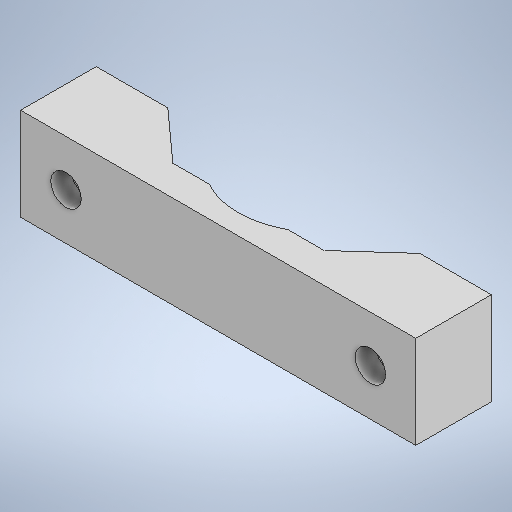
# Autodesk Inventor part: CameraTopSlider
Saved by Autodesk Inventor 2025.1 (Build 291241000, 241)
## iProperties
Created: 2026-04-27
Part Number: CameraTopSlider
Material: Generic
Document SubType Name: Modeling
Designer: User
Density: 1 g/cm^3
Appearance: Default
Author: User
## iProperties of the stored document CameraTopSlider_3DPrint.ipt
Created: 2026-04-30
Part Number: CameraTopSlider_3DPrint
Material: Generic
Document SubType Name: Modeling
Designer: User
Density: 1 g/cm^3
Appearance: Default
Author: User
Autodesk Inventor part; units mm, degrees
ref_plane "YZ Plane" through (0, 0, 0) normal (1, 0, 0) x (0, 1, 0)
ref_plane "XZ Plane" through (0, 0, 0) normal (0, 1, 0) x (-1, 0, 0)
ref_plane "XY Plane" through (0, 0, 0) normal (0, 0, 1) x (1, 0, 0)
sketch "Sketch1" plane through (0, 0, 0) normal (0, 0, 1) x (1, 0, 0)
  line L0 (-0.2, 0) -> (25.2, 0) projected
  line L1 (25.4, -1) -> (29.8, -1) projected
  line L2 (30, -0.8) -> (30, 3.8) projected
  line L3 (29.8, 4) -> (25.4, 4) projected
  line L4 (25.2, 3) -> (-0.2, 3) projected
  line L5 (-0.4, 4) -> (-4.8, 4) projected
  line L6 (-5, 3.8) -> (-5, -0.8) projected
  line L7 (-4.8, -1) -> (-0.4, -1) projected
  line L8 (25.1, -0.1) -> (-0.1, -0.1)
  line L9 (-0.1, -0.1) -> (-0.1, -1.1)
  line L10 (-0.1, -1.1) -> (-5.1, -1.1)
  line L11 (-5.1, -1.1) -> (-5.1, 4.1)
  line L12 (-5.1, 4.1) -> (-0.1, 4.1)
  line L13 (-0.1, 4.1) -> (-0.1, 3.1)
  line L14 (-0.1, 3.1) -> (25.1, 3.1)
  line L15 (25.1, 3.1) -> (25.1, 4.1)
  line L16 (25.1, 4.1) -> (30.1, 4.1)
  line L17 (30.1, 4.1) -> (30.1, -1.1)
  line L18 (30.1, -1.1) -> (25.1, -1.1)
  line L19 (25.1, -1.1) -> (25.1, -0.1)
  circle A0 centre (27.6, 1.5) radius 1.4 projected
  circle A1 centre (-2.6, 1.5) radius 1.4 projected
  line L20 (25.4, -1) -> (25.2, -0.8) projected
  line L21 (30, -0.8) -> (29.8, -1) projected
  line L22 (29.8, 4) -> (30, 3.8) projected
  line L23 (25.2, 3.8) -> (25.4, 4) projected
  line L24 (-0.4, 4) -> (-0.2, 3.8) projected
  line L25 (-5, 3.8) -> (-4.8, 4) projected
  line L26 (-4.8, -1) -> (-5, -0.8) projected
  line L27 (-0.2, -0.8) -> (-0.4, -1) projected
  line L28 (25.2, 3.8) -> (25.2, 3) projected
  line L29 (-0.2, 3) -> (-0.2, 3.8) projected
  line L30 (-0.2, -0.8) -> (-0.2, 0) projected
  line L31 (25.2, 0) -> (25.2, -0.8) projected
  point P0 (0, 0)
  dimension "d0" = 0.1
  constraints: 24 end point, 4 other
  measures "d0" distance between parallel lines of L0 L8
extrude "Extrusion1" add sketch "Sketch1" along normal blind 2 contours L30 L27 L7 L26 L6 L25 L5 L24 L29 L4 L28 L23 L3 L22 L2 L21 L1 L20 L31 L0 | L8 L9 L10 L11 L12 L13 L14 L15 L16 L17 L18 L19 | A0 | A1
sketch "Sketch2" plane through (0, 0, 2) normal (0, 0, 1) x (1, 0, 0)
  line L0 (25.1, -1.1) -> (30.1, -1.1) projected
  line L1 (30.1, -1.1) -> (30.1, 4.1) projected
  line L2 (30.1, 4.1) -> (25.1, 4.1) projected
  line L3 (25.1, 4.1) -> (25.1, 3.1) projected
  line L4 (25.1, 3.1) -> (-0.1, 3.1) projected
  line L5 (-0.1, 3.1) -> (-0.1, 4.1) projected
  line L6 (-0.1, 4.1) -> (-5.1, 4.1) projected
  line L7 (-5.1, 4.1) -> (-5.1, -1.1) projected
  line L8 (-5.1, -1.1) -> (-0.1, -1.1) projected
  line L9 (-0.1, -1.1) -> (-0.1, -0.1) projected
  line L10 (-0.1, -0.1) -> (25.1, -0.1) projected
  line L11 (25.1, -0.1) -> (25.1, -1.1) projected
  line L12 (-7.1, 6.1) -> (1.9, 6.1)
  line L13 (1.9, 6.1) -> (1.9, 5.1)
  line L14 (1.9, 5.1) -> (23.1, 5.1)
  line L15 (23.1, 5.1) -> (23.1, 6.1)
  line L16 (23.1, 6.1) -> (32.1, 6.1)
  line L17 (32.1, 6.1) -> (32.1, -3.1)
  line L18 (32.1, -3.1) -> (23.1, -3.1)
  line L19 (23.1, -3.1) -> (23.1, -2.1)
  line L20 (23.1, -2.1) -> (1.9, -2.1)
  line L21 (1.9, -2.1) -> (1.9, -3.1)
  line L22 (1.9, -3.1) -> (-7.1, -3.1)
  line L23 (-7.1, -3.1) -> (-7.1, 6.1)
  point P0 (0, 0)
  dimension "d3" = 2
  constraints: 24 end point, 11 other
  measures "d3" distance between parallel lines of L6 L12
ref_plane "Work Plane1" through (22.5, -3.5, -5.5) normal (0, 0, -1) x (0, 1, 0)
extrude "Extrusion2" add sketch "Sketch2" against normal up to surface (7.5 mm away)
sketch "Sketch3" plane through (1.9, -2.1, 2) normal (0, -1, 0) x (1, 0, 0)
  line L0 (6.9944, -4) -> (4.1, -4) projected
  arc A0 (8.2059, -3.4222) -> (6.9944, -4) centre (10.6, -10) ccw projected
  arc A1 (10.6, -3) -> (8.2059, -3.4222) centre (10.6, -10) ccw projected
  arc A2 (10.6, -3) -> (8.2059, -3.4222) centre (10.6, -10) ccw projected
  arc A3 (12.9941, -3.4222) -> (10.6, -3) centre (10.6, -10) ccw projected
  circle A4 centre (10.6, -10) radius 5.6 projected
  arc A5 (14.2056, -4) -> (12.9941, -3.4222) centre (10.6, -10) ccw projected
  line L1 (17.1, -4) -> (14.2056, -4) projected
  line L2 (17.1, -7.4019) -> (17.1, -4) projected
  line L3 (4.1, -4) -> (4.1, -7.4019) projected
  circle A6 centre (10.6, -10) radius 5.6 projected
  arc A7 (4.1, -7.4019) -> (3.8918, -8) centre (10.6, -10) ccw projected
  arc A8 (17.3082, -8) -> (17.1, -7.4019) centre (10.6, -10) ccw projected
  arc A9 (7.8638, -2.4825) -> (6.727, -3) centre (10.6, -10) ccw
  line L4 (6.727, -3) -> (3.1, -3)
  line L5 (3.1, -3) -> (3.1, -7.2161)
  arc A10 (3.1, -7.2161) -> (2.9335, -7.7143) centre (10.6, -10) ccw
  arc A11 (10.6, -2) -> (7.8638, -2.4825) centre (10.6, -10) ccw
  arc A12 (13.3362, -2.4825) -> (10.6, -2) centre (10.6, -10) ccw
  arc A13 (14.473, -3) -> (13.3362, -2.4825) centre (10.6, -10) ccw
  line L6 (14.473, -3) -> (18.1, -3)
  line L7 (18.1, -3) -> (18.1, -7.2161)
  arc A14 (18.2665, -7.7143) -> (18.1, -7.2161) centre (10.6, -10) ccw
  line L8 (0, -7.5) -> (21.2, -7.5) projected
  point P0 (-1.9, -2)
  point P1 (17.1383, -7.5)
  point P2 (18.1993, -7.5)
  point P3 (10.6, -2)
  point P4 (7.8638, -2.4825)
  point P5 (3.0007, -7.5)
  point P6 (4.0617, -7.5)
  dimension "d6" = 1
  dimension "d7" = 1
  dimension "d8" = 1
  constraints: 12 point on circle, 8 end point, 6 centre point, 7 other
  measures "d6" radial gap between concentric circles of A0 A9
  measures "d7" radial gap between concentric circles of A1 A11
  measures "d8" radial gap between concentric circles of A3 A12
extrude "Extrusion3" cut sketch "Sketch3" against normal blind 10 contours A0 A1 A3 A5 L1 L2 A8 L8 A4 A7 L3 L0 | L0 L3 A7 L8 A10 L5 L4 A9 A11 A12 A13 L6 L7 A14 A8 L2 L1 A5 A3 A1 A0 | A4 L8 picked at (9.9261, -6.5925)
sketch "Sketch4" plane through (1.9, -2.1, 2) normal (0, -1, 0) x (1, 0, 0)
  line L0 (3.1, -7.2161) -> (3.1, -3) projected
  line L1 (0, -7.5) -> (3.0007, -7.5) projected
  line L2 (-9, -7.5) -> (0, -7.5) projected
  line L3 (-1.9, -6.3) -> (-1.9, -15) projected
  line L4 (18.1, -3) -> (18.1, -7.2161) projected
  arc A0 (3.1, -7.2161) -> (3.0007, -7.5) centre (10.6, -10) ccw projected
  arc A1 (18.1993, -7.5) -> (18.1, -7.2161) centre (10.6, -10) ccw projected
  line L5 (18.1993, -7.5) -> (21.2, -7.5) projected
  line L6 (21.2, -7.5) -> (30.2, -7.5) projected
  line L7 (23.1, -15) -> (23.1, -6.3) projected
  line L8 (3.1, -3) -> (-1.9, -7.5)
  line L9 (18.1, -3) -> (14.473, -3) projected
  line L10 (18.1, -3) -> (23.1, -7.5)
  point P0 (-1.9, -2)
  constraints: 4 end point, 4 point on line
extrude "Extrusion4" cut sketch "Sketch4" along normal mid plane 33.75
sketch "Sketch5" plane through (0, 0, 2) normal (0, 0, 1) x (1, 0, 0)
  line L0 (-2, -1) -> (-4.8, -1) projected
  line L1 (-5, -0.8) -> (-5, 3.8) projected
  line L2 (-4.8, 4) -> (-2, 4) projected
  line L3 (27, 4) -> (29.8, 4) projected
  line L4 (30, 3.8) -> (30, -0.8) projected
  line L5 (29.8, -1) -> (27, -1) projected
  line L6 (25.2, 4) -> (30, -1)
  line L7 (-0.2, 4) -> (-5, -1)
  circle A0 centre (-2.6, 1.5) radius 1.5
  circle A1 centre (27.6, 1.5) radius 1.5
  line L8 (30, 3.8) -> (29.8, 4) projected
  line L9 (29.8, -1) -> (30, -0.8) projected
  line L10 (-5, -0.8) -> (-4.8, -1) projected
  line L11 (-4.8, 4) -> (-5, 3.8) projected
  arc A2 (-2, 2.7649) -> (-2, 0.2351) centre (-2.6, 1.5) ccw projected
  line L12 (-2, 2.7649) -> (-2, 4) projected
  line L13 (-2, -1) -> (-2, 0.2351) projected
  arc A3 (27, 0.2351) -> (27, 2.7649) centre (27.6, 1.5) ccw projected
  line L14 (27, 0.2351) -> (27, -1) projected
  line L15 (27, 4) -> (27, 2.7649) projected
  dimension "d13" = 3
  dimension "d14" = 3
  constraints: 4 end point, 2 centre point, 2 midpoint
  measures "d13" diameter of A0
  measures "d14" diameter of A1
extrude "Extrusion5" cut sketch "Sketch5" against normal blind 33.75 contours L13 A2 L7 A0 | A0 L7 A2 L13 | A0 L12 A2 L7 | A2 L12 A0 L7 | L15 A3 L6 A1 | A1 L6 A3 L15 | L6 A3 L14 A1 | A1 L14 A3 L6
chamfer "Chamfer1" distance 0.2 angle 45 4 edges at (25.1, 3.1, -2.75) (25.1, -0.1, -2.75) (-0.1, -0.1, -2.75) (-0.1, 3.1, -2.75)
sketch "Sketch6" plane through (16.373, 3.1, -1) normal (0, -1, 0) x (1, 0, 0)
  line L0 (8.527, 1) -> (8.527, -4.41) projected
  line L1 (8.527, 1) -> (-3.873, 1) projected
  arc A0 (0, 0) -> (-3.873, 1) centre (-3.873, -7) ccw projected
  line L2 (0, 0) -> (3.627, 0) projected
  line L3 (3.627, 0) -> (8.527, -4.41) projected
  line L4 (8.627, -4.5) -> (8.727, -4.5) projected
  line L5 (8.727, -4.5) -> (8.727, 1) projected
  line L6 (8.727, 1) -> (8.527, 1) projected
  line L7 (8.527, 1) -> (8.527, -4.41) projected
  line L8 (8.527, -4.41) -> (8.627, -4.5) projected
  line L9 (8.727, 1) -> (8.727, -4.5) projected
  line L10 (-16.273, -4.41) -> (-16.273, 1) projected
  line L11 (-16.273, -4.41) -> (-11.373, 0) projected
  line L12 (-11.373, 0) -> (-7.746, 0) projected
  arc A1 (-3.873, 1) -> (-7.746, 0) centre (-3.873, -7) ccw projected
  line L13 (-3.873, 1) -> (-16.273, 1) projected
  line L14 (-16.373, -4.5) -> (-16.273, -4.41) projected
  line L15 (-16.273, -4.41) -> (-16.273, 1) projected
  line L16 (-16.273, 1) -> (-16.473, 1) projected
  line L17 (-16.473, 1) -> (-16.473, -4.5) projected
  line L18 (-16.473, -4.5) -> (-16.373, -4.5) projected
  point P0 (-16.373, 1)
  point P1 (-3.873, 1)
  point P2 (-3.873, 1)
  point P3 (-3.873, 1)
  point P4 (-3.873, 1)
  point P5 (8.527, 1)
extrude "Extrusion6" cut sketch "Sketch6" against normal up to surface (1 mm away)
sketch "Sketch7" plane through (16.373, -0.1, -1) normal (0, 1, 0) x (1, 0, 0)
  line L0 (-16.273, -1) -> (-16.273, 4.41) projected
  line L1 (-16.273, -1) -> (-3.873, -1) projected
  arc A0 (-7.746, 0) -> (-3.873, -1) centre (-3.873, 7) ccw projected
  line L2 (-7.746, 0) -> (-11.373, 0) projected
  line L3 (-11.373, 0) -> (-16.273, 4.41) projected
  line L4 (-16.373, 4.5) -> (-16.473, 4.5) projected
  line L5 (-16.473, 4.5) -> (-16.473, -1) projected
  line L6 (-16.473, -1) -> (-16.273, -1) projected
  line L7 (-16.273, -1) -> (-16.273, 4.41) projected
  line L8 (-16.273, 4.41) -> (-16.373, 4.5) projected
  line L9 (8.527, 4.41) -> (8.527, -1) projected
  line L10 (8.527, 4.41) -> (3.627, 0) projected
  line L11 (3.627, 0) -> (0, 0) projected
  arc A1 (-3.873, -1) -> (0, 0) centre (-3.873, 7) ccw projected
  line L12 (-3.873, -1) -> (8.527, -1) projected
  line L13 (8.627, 4.5) -> (8.527, 4.41) projected
  line L14 (8.527, 4.41) -> (8.527, -1) projected
  line L15 (8.527, -1) -> (8.727, -1) projected
  line L16 (8.727, -1) -> (8.727, 4.5) projected
  line L17 (8.727, 4.5) -> (8.627, 4.5) projected
  point P0 (-16.373, -1)
extrude "Extrusion7" cut sketch "Sketch7" against normal up to surface (1 mm away)
sketch "Sketch8" plane through (1.9, -2.1, 2) normal (0, -1, 0) x (1, 0, 0)
  line L0 (18.1, -3) -> (21.2, -5.79) projected
  line L1 (21.2, 0) -> (21.2, -5.79) projected
  line L2 (0, 0) -> (21.2, 0) projected
  line L3 (0, 0) -> (0, -5.79) projected
  line L4 (0, -5.79) -> (3.1, -3) projected
  line L5 (3.1, -3) -> (6.727, -3) projected
  arc A0 (14.473, -3) -> (6.727, -3) centre (10.6, -10) ccw projected
  line L6 (14.473, -3) -> (18.1, -3) projected
  point P0 (-1.9, -2)
extrude "Extrusion8" add sketch "Sketch8" along normal up to surface (1 mm away)
sketch "Sketch9" plane through (1.9, 5.1, 2) normal (0, 1, 0) x (1, 0, 0)
  line L0 (21.2, 5.79) -> (18.1, 3) projected
  line L1 (18.1, 3) -> (14.473, 3) projected
  arc A0 (6.727, 3) -> (14.473, 3) centre (10.6, 10) ccw projected
  line L2 (6.727, 3) -> (3.1, 3) projected
  line L3 (3.1, 3) -> (0, 5.79) projected
  line L4 (0, 0) -> (0, 5.79) projected
  line L5 (21.2, 0) -> (0, 0) projected
  line L6 (21.2, 0) -> (21.2, 5.79) projected
  point P0 (-1.9, 2)
extrude "Extrusion9" add sketch "Sketch9" along normal up to surface (1 mm away)
sketch "Sketch10" plane through (32.1, -3.1, -5.5) normal (0, 0, -1) x (-1, 0, 0)
  line L0 (37.2, 2) -> (19.6, 2) projected
  line L1 (37.2, 7.2) -> (37.2, 2) projected
  line L2 (37.2, 7.2) -> (19.6, 7.2) projected
  line L3 (2, 7.2) -> (19.6, 7.2) projected
  line L4 (2, 2) -> (2, 7.2) projected
  line L5 (19.6, 2) -> (2, 2) projected
  circle A0 centre (34.7, 4.6) radius 1.5 projected
  circle A1 centre (4.5, 4.6) radius 1.5 projected
  line L6 (19.6, 7.4) -> (37.4, 7.4)
  line L7 (37.4, 7.4) -> (37.4, 1.8)
  line L8 (37.4, 1.8) -> (19.6, 1.8)
  line L9 (19.6, 1.8) -> (1.8, 1.8)
  line L10 (1.8, 1.8) -> (1.8, 7.4)
  line L11 (1.8, 7.4) -> (19.6, 7.4)
  point P0 (32.1, 3.1)
  dimension "d28" = 0.2
  constraints: 12 end point, 5 other
  measures "d28" distance between parallel lines of L3 L11
extrude "Extrusion10" cut sketch "Sketch10" against normal up to surface (5.5 mm away) contours L0 L5 L4 L3 L2 L1 | A0 | A1 | L6 L7 L8 L9 L10 L11
body "Solid1"
